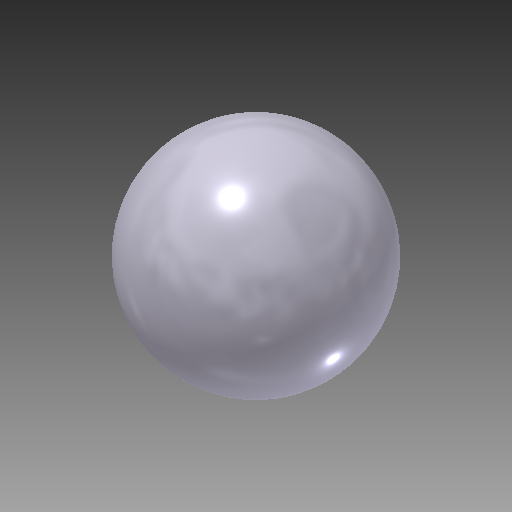
# Autodesk Inventor part: sapphire ball
Saved by Autodesk Inventor 2017 (Build 210142000, 142)
## iProperties
Created: 2009-05-06
Part Number: sapphire ball
Document SubType Name: Modeling
Designer: Serena
Material: Generic
Density: 1 g/cm^3
Appearance: Opal
Author: Serena
Autodesk Inventor part; units mm, degrees
ref_plane "YZ Plane" through (0, 0, 0) normal (1, 0, 0) x (0, 1, 0)
ref_plane "XZ Plane" through (0, 0, 0) normal (0, 1, 0) x (-1, 0, 0)
ref_plane "XY Plane" through (0, 0, 0) normal (0, 0, 1) x (1, 0, 0)
sketch "Sketch1" plane through (0, 0, 0) normal (0, 0, 1) x (1, 0, 0)
  circle A0 centre (0, 0) radius 1
  line L0 (0, 0) -> (1, 0)
  line L1 (0, 0) -> (0, -1)
  arc A1 (0, -1) -> (1, 0) centre (0, 0) ccw
  line L2 (0, 0) -> (-1, 0)
  line L3 (0, 0) -> (0, 1)
  arc A2 (0, 1) -> (-1, 0) centre (0, 0) ccw
  dimension "d0" = 2
  constraints: 8 end point, 8 point on circle, 3 centre point, 3 perpendicular, 2 concentric, 1 horizontal
  measures "d0" diameter of A0
revolve "Revolution1" add sketch "Sketch1" angle 360 about axis through (0, 0, 0) along (0, -1, 0) contours A0 L1 L0
sketch "Sketch2" plane through (0, 0, 0) normal (0, 0, 1) x (1, 0, 0)
  circle A0 centre (0, 0) radius 1
  line L0 (0, 0) -> (1, 0)
  line L1 (0, 0) -> (0, 1)
  arc A1 (1, 0) -> (0, 1) centre (0, 0) ccw
  dimension "d2" = 2
  constraints: 4 end point, 4 point on circle, 2 centre point, 1 concentric, 1 horizontal, 1 perpendicular
  measures "d2" diameter of A0
revolve "Revolution2" add sketch "Sketch2" angle 360 about axis through (0, 0, 0) along (0, 1, 0) picked at (0.0742, 0.6583) contours L0 L1 A0
body "Solid1"
